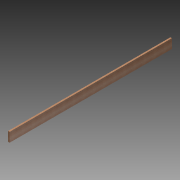
# Autodesk Inventor part: Ledger Board
Saved by Autodesk Inventor 2015 (Build 190159000, 159)
## iProperties
Created: 2014-05-27
Part Number: Ledger Board
Material: Wood (Birch)
Document SubType Name: Modeling
Designer: Haden
Density: 0.55 g/cm^3
Appearance: Birch - Natural Polished
Mass: 20008.6 g
Surface Area: 22372.5 cm^2
Volume: 36379.3 cm^3
Author: Haden
Autodesk Inventor part; units mm, degrees
ref_plane "YZ Plane" through (0, 0, 0) normal (1, 0, 0) x (0, 1, 0)
ref_plane "XZ Plane" through (0, 0, 0) normal (0, 1, 0) x (-1, 0, 0)
ref_plane "XY Plane" through (0, 0, 0) normal (0, 0, 1) x (1, 0, 0)
sketch "Sketch1" plane through (0, 0, 0) normal (0, 0, 1) x (1, 0, 0)
  line L0 (0, 0) -> (38.1, 0)
  line L1 (38.1, 0) -> (38.1, -234.95)
  line L2 (38.1, -234.95) -> (0, -234.95)
  line L3 (0, -234.95) -> (0, 0)
  dimension "d0" = 234.95
  dimension "d1" = 38.1
  constraints: 8 end point, 2 parallel, 1 horizontal, 1 perpendicular
  measures "d0" distance of L0.end L1.end
  measures "d1" distance of L1.end L2.end
extrude "Extrusion1" add sketch "Sketch1" along normal blind 4064
body "Solid1"
